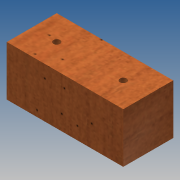
# Autodesk Inventor part: hubjig_spacer
Saved by Autodesk Inventor 2014 SP1 (Build 180222100, 222)
## iProperties
Created: 2014-08-29
Part Number: hubjig_spacer
Material: Wood (Cherry)
Document SubType Name: Modeling
Designer: Dave
Mass: 80.3176 g
Surface Area: 175.919 cm^2
Volume: 127.488 cm^3
Density: 0.63 g/cm^3
Appearance: Cherry - Natural Low Gloss
Author: Dave
Autodesk Inventor part; units mm, degrees
ref_plane "YZ Plane" through (0, 0, 0) normal (1, 0, 0) x (0, 1, 0)
ref_plane "XZ Plane" through (0, 0, 0) normal (0, 1, 0) x (-1, 0, 0)
ref_plane "XY Plane" through (0, 0, 0) normal (0, 0, 1) x (1, 0, 0)
sketch "Sketch1" plane through (0, 0, 0) normal (0, 0, 1) x (1, 0, 0)
  line L0 (0, 0) -> (88.9, 0)
  line L1 (88.9, 0) -> (88.9, 38.1)
  line L2 (88.9, 38.1) -> (0, 38.1)
  line L3 (0, 38.1) -> (0, 0)
  dimension "d0" = 88.9
  dimension "d1" = 38.1
  constraints: 8 end point, 2 parallel, 1 horizontal, 1 perpendicular
  measures "d0" distance of L0.start L0.end
  measures "d1" distance of L2.end L0.start
extrude "Extrusion1" add sketch "Sketch1" along normal blind 38.1
sketch "Sketch2" plane through (0, 38.1, 0) normal (0, 1, 0) x (1, 0, 0)
  line L0 (88.9, 0) -> (0, 0) projected
  line L1 (0, 0) -> (0, -38.1) projected
  line L2 (88.9, -38.1) -> (0, -38.1) projected
  circle A0 centre (19.05, -19.05) radius 5.8141
  circle A1 centre (69.85, -19.05) radius 5.8141
  dimension "d4" = 19.05
  dimension "d5" = 19.05
  dimension "d8" = 50.8
  constraints: 2 centre point, 1 horizontal, 2 other
  measures "d4" distance from line of L2 A0.centre
  measures "d5" distance from line of L1 A0.centre
  measures "d8" distance of A0.centre A1.centre
hole "Hole1" at (19.05, 38.1, 19.05) at (69.85, 38.1, 19.05) direction (0, -1, 0) diameter 5.1054 end through all clearance for "Flat Head Machine Screw (82)" size "#10" standard "Ansi Unified Screw Threads"
equation "\"d18\" = d8"
body "Solid1"
